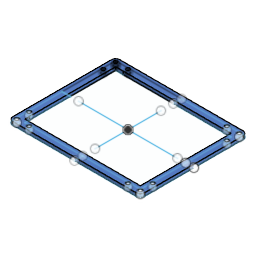
SLAM_Rescue_Chassis design (Autodesk Fusion 360 archive; units mm, degrees)
design "center"
Autodesk Fusion 360 part; units mm, degrees
sketch "Sketch1" plane through (0, 0, 0) normal (0, 0, 1) x (1, 0, 0)
  circle A0 centre (-75, 60) radius 2.1
  circle A1 centre (-60, 60) radius 2.1
  circle A2 centre (-75, 45) radius 2.1
  line L0 (-75, 65) -> (0, 65)
  line L1 (0, 65) -> (0, 55)
  line L2 (0, 55) -> (-60.788, 55)
  line L3 (-70, 49.6316) -> (-70, 0)
  line L4 (-70, 0) -> (-80, 0)
  line L5 (-80, 0) -> (-80, 60)
  arc A3 (-75, 65) -> (-80, 60) centre (-75, 60) ccw
  line L6 (0, 40) -> (0, -40)
  line L7 (-60, 0) -> (60, 0)
  line L8 (-70, -49.6316) -> (-70, 0)
  line L9 (0, -55) -> (-60.788, -55)
  line L10 (-75, -65) -> (0, -65)
  line L11 (-80, 0) -> (-80, -60)
  arc A4 (-80, -60) -> (-75, -65) centre (-75, -60) ccw
  circle A5 centre (-75, -60) radius 2.1
  circle A6 centre (-60, -60) radius 2.1
  circle A7 centre (-75, -45) radius 2.1
  line L12 (-70, 0) -> (-80, 0)
  line L13 (0, -65) -> (0, -55)
  line L14 (80, 0) -> (80, -60)
  line L15 (70, -49.6316) -> (70, 0)
  circle A8 centre (75, -60) radius 2.1
  circle A9 centre (60, -60) radius 2.1
  circle A10 centre (75, -45) radius 2.1
  line L16 (75, -65) -> (0, -65)
  arc A11 (75, -65) -> (80, -60) centre (75, -60) ccw
  line L17 (0, -55) -> (60.788, -55)
  line L18 (70, 49.6316) -> (70, 0)
  line L19 (80, 0) -> (80, 60)
  line L20 (0, 55) -> (60.788, 55)
  line L21 (75, 65) -> (0, 65)
  circle A12 centre (75, 60) radius 2.1
  arc A13 (80, 60) -> (75, 65) centre (75, 60) ccw
  circle A14 centre (75, 45) radius 2.1
  circle A15 centre (60, 60) radius 2.1
  line L22 (-70, 49.6316) -> (-70, 55)
  line L23 (-70, 55) -> (-60.788, 55)
  line L24 (-70, -55) -> (-60.788, -55)
  line L25 (-70, -55) -> (-70, -49.6316)
  line L26 (60.788, -55) -> (70, -55)
  line L27 (70, -55) -> (70, -49.6316)
  line L28 (60.788, 55) -> (70, 55)
  line L29 (70, 49.6316) -> (70, 55)
  dimension "d1" = 4.2
  dimension "d2" = 4.2
  dimension "d3" = 4.2
  dimension "d4" = 15
  dimension "d5" = 15
  dimension "d6" = 75
  dimension "d7" = 60
  dimension "d8" = 10
  constraint concentric A0 A3
  constraint tangent L0 A3
  constraint horizontal L0
  constraint perpendicular L0 L1
  constraint tangent L2 A3
  constraint perpendicular L1 L2
  constraint tangent L3 A3
  constraint perpendicular L0 L3
  constraint perpendicular L3 L4
  constraint tangent L5 A3
  constraint perpendicular L4 L5
  constraint horizontal A1.centre A0.centre
  constraint vertical A0.centre A2.centre
  constraint midpoint L6 origin
  constraint vertical L6
  constraint midpoint L7 origin
  constraint perpendicular L6 L7
  constraint symmetric A0 L7 A5
  constraint symmetric A1 L7 A6
  constraint symmetric A2 L7 A7
  constraint symmetric L0.start L7 L10.start
  constraint symmetric L0.end L7 L10.end
  constraint symmetric L1.end L7 L9.start
  constraint symmetric L3.end L7 L4.start
  constraint symmetric L4.end L7 L5.start
  constraint symmetric L5.end L7 L11.end
  constraint symmetric A3 L7 A4
  constraint symmetric L3.start L7 L8.start
  constraint symmetric L2.end L7 L9.end
  constraint symmetric A0 L6 A12
  constraint symmetric A1 L6 A15
  constraint symmetric A2 L6 A14
  constraint symmetric L0.start L6 L21.start
  constraint symmetric L0.end L6 L1.start
  constraint symmetric L1.end L6 L2.start
  constraint symmetric L3.end L6 L15.end
  constraint symmetric L4.end L6 L14.start
  constraint symmetric L5.end L6 L19.end
  constraint symmetric A3 L6 A13
  constraint symmetric L3.start L6 L18.start
  constraint symmetric L2.end L6 L20.end
  constraint symmetric L6 L9.end L17.end
  constraint symmetric L6 L8.start L15.start
  constraint symmetric L6 L3.end L15.end
  constraint symmetric L6 L9.start L13.end
  constraint symmetric L6 L10.start L16.start
  constraint symmetric L6 L10.end L13.start
  constraint symmetric L6 L4.end L14.start
  constraint symmetric L6 L11.end L14.end
  constraint symmetric L6 A4 A11
  constraint symmetric L6 A5 A8
  constraint symmetric L6 A6 A9
  constraint symmetric L6 A7 A10
  constraint parallel L3 L22
  constraint perpendicular L25 L26
  constraint perpendicular L26 L27
  constraint parallel L20 L28
  constraint perpendicular L28 L29
  measures "d1" diameter of A0
  measures "d2" diameter of A1
  measures "d3" diameter of A2
  measures "d4" distance of A0.centre A2.centre
  measures "d5" distance of A0.centre A1.centre
  measures "d6" horizontal distance of origin A0.centre
  measures "d7" vertical distance of origin A0.centre
  measures "d8" diameter of A3
extrude "Extrude3" add sketch "Sketch1" along normal blind 3.75 contours L0 L1 L2 L3 L4 L5 A3 L12 L22 L23 | L1 L13 L14 L15 L16 A11 L17 L18 L19 L20 L21 A13 L26 L27 L28 L29 | L4 L8 L9 L10 L11 A4 L12 L13 L24 L25

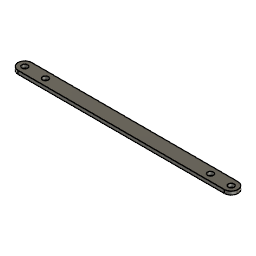
design "side"
Autodesk Fusion 360 part; units mm, degrees
sketch "Sketch1" plane through (0, 0, 0) normal (0, 0, 1) x (1, 0, 0)
  circle A0 centre (-60, 0) radius 2.1
  circle A1 centre (-75, 0) radius 2.1
  circle A2 centre (60, 0) radius 2.1
  circle A3 centre (75, 0) radius 2.1
  line L0 (-75, 5) -> (75, 5)
  line L1 (-75, -5) -> (75, -5)
  arc A4 (-75, 5) -> (-75, -5) centre (-75, 0) ccw
  arc A5 (75, -5) -> (75, 5) centre (75, 0) ccw
  dimension "d1" = 4.2
  dimension "d2" = 4.2
  dimension "d3" = 4.2
  dimension "d4" = 4.2
  dimension "d7" = 75
  dimension "d9" = 15
  dimension "d11" = 75
  dimension "d12" = 15
  dimension "d13" = 10
  dimension "d14" = 10
  constraint horizontal A0.centre A1.centre
  constraint horizontal origin A0.centre
  constraint horizontal origin A2.centre
  constraint horizontal A2.centre A3.centre
  constraint concentric A1 A4
  constraint concentric A3 A5
  constraint tangent L0 A5
  constraint horizontal L0
  constraint tangent L1 A5
  constraint parallel L0 L1
  measures "d1" diameter of A3
  measures "d2" diameter of A2
  measures "d3" diameter of A1
  measures "d4" diameter of A0
  measures "d7" distance of origin A1.centre
  measures "d9" distance of A0.centre A1.centre
  measures "d11" distance of origin A3.centre
  measures "d12" distance of A2.centre A3.centre
  measures "d13" diameter of A4
  measures "d14" diameter of A5
extrude "Extrude1" add sketch "Sketch1" along normal blind 2.5
